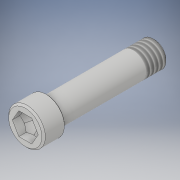
# Autodesk Inventor part: WkretDoNapinacza
Saved by Autodesk Inventor 2019 (Build 230136000, 136)
## iProperties
Created: 2020-08-27
Part Number: WkretDoNapinacza
Material: Generic
Document SubType Name: Modeling
Designer: estee
Density: 1 g/cm^3
Appearance: Default
Author: estee
Autodesk Inventor part; units mm, degrees
ref_plane "YZ Plane" through (0, 0, 0) normal (1, 0, 0) x (0, 1, 0)
ref_plane "XZ Plane" through (0, 0, 0) normal (0, 1, 0) x (-1, 0, 0)
ref_plane "XY Plane" through (0, 0, 0) normal (0, 0, 1) x (1, 0, 0)
sketch "Sketch1" plane through (0, 0, 0) normal (1, 0, 0) x (0, 1, 0)
  line L0 (0, 0) -> (4.25, 0)
  line L1 (4.25, 0) -> (4.25, -5)
  line L2 (4.25, -5) -> (3, -5)
  line L3 (3, -5) -> (3, -30)
  line L4 (3, -30) -> (0, -30)
  line L5 (0, 0) -> (0, -30)
  line L6 (0, -36) -> (0, 6) projected
  dimension "d0" = 4.25
  dimension "d1" = 1.25
  dimension "d2" = 5
  dimension "d3" = 25
  constraints: 12 end point, 4 perpendicular, 1 horizontal, 1 vertical
  measures "d0" distance of L0.start L0.end
  measures "d1" distance of L1.end L2.end
  measures "d2" distance of L0.end L1.end
  measures "d3" distance of L2.end L3.end
revolve "Revolution1" add sketch "Sketch1" angle 360 about axis through (0, 0, -10) along (0, 0, 1)
thread "Thread1" size "M6x1" class "6g" standard "ANSI Metric M Profile" length 5
sketch "Sketch2" plane through (0, 0, 0) normal (0, 0, 1) x (1, 0, 0)
  circle A0 centre (0, 0) radius 3 projected
  line L0 (-3, -0.0001) -> (-1.4999, 2.5981)
  line L1 (-1.4999, 2.5981) -> (1.4999, 2.5981)
  line L2 (1.4999, 2.5981) -> (3, -0.0001)
  line L3 (3, -0.0001) -> (1.5001, -2.598)
  line L4 (1.5001, -2.598) -> (-1.5001, -2.598)
  line L5 (-1.5001, -2.598) -> (-3, -0.0001)
  dimension "d7" = 120
  dimension "d8" = 120
  constraints: 12 end point, 6 point on circle, 3 parallel, 1 horizontal, 1 point on line
  measures "d7" angle of L5 L0
  measures "d8" angle of L1 L0
extrude "Extrusion1" cut sketch "Sketch2" against normal blind 4.5 contours L3 L4 L5 L0 L1 L2
chamfer "Chamfer1" distance 2.5 angle 45 6 edges at (2.25, 1.299, -4.5) (0, 2.5981, -4.5) (-2.25, 1.299, -4.5) (2.25, -1.2991, -4.5) (0, -2.598, -4.5) (-2.25, -1.2991, -4.5)
fillet "Fillet1" radius 3.5 6 edges at (-0.7782, 1.3481, -3.25) (-1.5566, -0.0001, -3.25) (0.7782, 1.3481, -3.25) (1.5566, -0.0001, -3.25) (0.7784, -1.348, -3.25) (-0.7784, -1.348, -3.25)
chamfer "Chamfer2" distance 0.2 angle 45 1 edges at (0, -4.25, -5)
chamfer "Chamfer3" distance 0.4 angle 45 2 edges at (0, -4.25, 0) (0, -3, -30)
body "Solid1"
